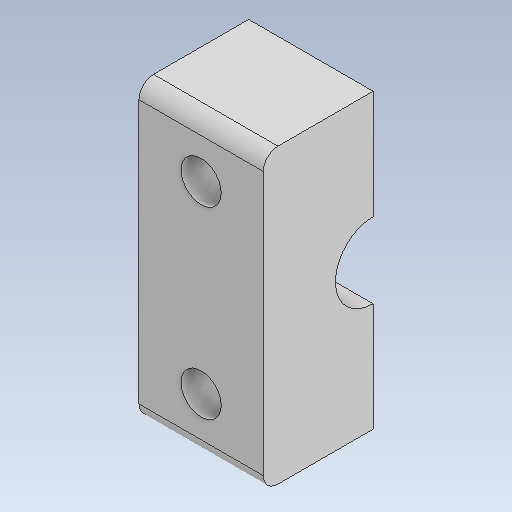
# Autodesk Inventor part: 0008-10-010 Fixare AxaX
Saved by Autodesk Inventor 2020 (Build 240168000, 168)
## iProperties
Created: 2021-02-27
Part Number: 0008-10-010 Fixare AxaX
Material: Generic
Document SubType Name: Modeling
Designer: Iulian Bors
Density: 1 g/cm^3
Appearance: Default
Description: Fixare Axa
Mass: 8.74982 g
Surface Area: 34.7733 cm^2
Volume: 8.74982 cm^3
Author: Iulian Bors
Subject: 010
Autodesk Inventor part; units mm, degrees
ref_plane "YZ Plane" through (0, 0, 0) normal (1, 0, 0) x (0, 1, 0)
ref_plane "XZ Plane" through (0, 0, 0) normal (0, 1, 0) x (-1, 0, 0)
ref_plane "XY Plane" through (0, 0, 0) normal (0, 0, 1) x (1, 0, 0)
sketch "Sketch1" plane through (0, 0, 0) normal (0, 0, 1) x (1, 0, 0)
  line L0 (-8.5, 20) -> (8.5, 20)
  line L1 (8.5, 20) -> (8.5, -20)
  line L2 (8.5, -20) -> (-8.5, -20)
  line L3 (-8.5, -20) -> (-8.5, 20)
  point P0 (0, 0)
  point P1 (-8.5, 0)
  point P2 (0, 20)
  dimension "d0" = 40
  dimension "d1" = 17
  constraints: 8 end point, 2 midpoint, 2 parallel, 1 horizontal, 1 horizontal alignment, 1 perpendicular, 1 vertical alignment
  measures "d0" distance of L2.end L0.start
  measures "d1" distance of L0.start L0.end
extrude "Extrusion1" add sketch "Sketch1" along normal blind 15
sketch "Sketch2" plane through (-8.5, -20, 0) normal (-1, 0, 0) x (0, 0, 1)
  circle A0 centre (0, 20) radius 5.15
  line L0 (0, 40) -> (0, 0) projected
  dimension "d5" = 10.3
  dimension "d8" = 0
  constraints: 1 centre point, 1 coincident, 1 midpoint
  measures "d5" diameter of A0
  measures "d8" distance of point (0, 20) A0.centre
extrude "Extrusion2" cut sketch "Sketch2" against normal through all
sketch "Sketch3" plane through (0, 0, 0) normal (0, 0, -1) x (-1, 0, 0)
  line L0 (-8.5, 5.15) -> (-8.5, 20) projected
  line L1 (-8.5, -20) -> (-8.5, -5.15) projected
  line L2 (8.5, -20) -> (-8.5, -20) projected
  line L3 (-8.5, 20) -> (8.5, 20) projected
  point P0 (0, 0)
  point P1 (0, -12.575)
  point P2 (0, 12.575)
  point P3 (-8.5, 12.575)
  point P4 (-8.5, -12.575)
  point P5 (0, -20)
  point P6 (0, 20)
  constraints: 4 midpoint, 2 horizontal alignment, 2 vertical alignment
hole "Hole1" at (0, -12.575, 0) at (0, 12.575, 0) direction (0, 0, 1) diameter 5.5 end through all
fillet "Fillet1" radius 2 2 edges at (0, -20, 15) (0, 20, 15)
body "Solid1"
